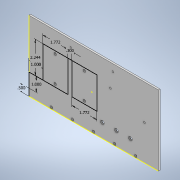
# Autodesk Inventor part: sheetmetalback2.0
Saved by Autodesk Inventor 2020.2 (Build 242310000, 310)
## iProperties
Created: 2020-02-06
Part Number: sheetmetalback2.0
Material: Generic
Document SubType Name: Sheet Metal
Designer: ColinP
Density: 1 g/cm^3
Sheet Metal Rule: Default
Appearance: Default
Author: ColinP
Autodesk Inventor part; units mm, degrees
ref_plane "YZ Plane" through (0, 0, 0) normal (1, 0, 0) x (0, 1, 0)
ref_plane "XZ Plane" through (0, 0, 0) normal (0, 1, 0) x (-1, 0, 0)
ref_plane "XY Plane" through (0, 0, 0) normal (0, 0, 1) x (1, 0, 0)
sketch "Sketch1" plane through (0, 0, 0) normal (0, 0, 1) x (1, 0, 0)
  line L0 (120.396, 63.5) -> (-114.3, 63.5)
  line L1 (-114.3, 63.5) -> (-114.3, -63.5)
  line L2 (-114.3, -63.5) -> (120.396, -63.5)
  line L3 (120.396, -63.5) -> (120.396, 63.5)
  point P0 (0, 0)
  dimension "d0" = 234.696
  dimension "d1" = 127
  measures "d0" distance of L2.end L1.end
  measures "d1" distance of L1.end L0.end
extrude "Plate1" add sketch "Sketch1" along normal blind 3.048
sketch "Sketch2" plane through (0, 0, 3.048) normal (0, 0, 1) x (1, 0, 0)
  line L0 (-114.3, 63.5) -> (-114.3, -63.5) projected
  line L1 (-114.3, -63.5) -> (-114.3, -60.325)
  line L2 (-114.3, -60.325) -> (-73.152, -60.325)
  line L3 (-73.152, -60.325) -> (-35.052, -60.325)
  line L4 (-35.052, -60.325) -> (3.048, -60.325)
  line L5 (3.048, -60.325) -> (41.148, -60.325)
  line L6 (41.148, -60.325) -> (79.248, -60.325)
  line L7 (79.248, -60.325) -> (120.396, -60.325)
  line L8 (120.396, -63.5) -> (120.396, 63.5) projected
  point P0 (0, 0)
  dimension "d3" = 3.175
  dimension "d4" = 41.148
  dimension "d5" = 38.1
  dimension "d6" = 38.1
  dimension "d7" = 38.1
  dimension "d8" = 38.1
  constraints: 14 end point, 6 point on line, 1 horizontal, 1 perpendicular
  measures "d3" distance of L0.end L1.end
  measures "d4" distance of L1.end L2.end
  measures "d5" distance of L2.end L3.end
  measures "d6" distance of L3.end L4.end
  measures "d7" distance of L4.end L5.end
  measures "d8" distance of L5.end L6.end
hole "Hole1" at (-73.152, -60.325, 3.048) at (-35.052, -60.325, 3.048) at (3.048, -60.325, 3.048) at (41.148, -60.325, 3.048) at (79.248, -60.325, 3.048) direction (0, 0, -1) diameter 4.4958 depth 3.048 clearance for "Hex Machine Screw" size "#8" standard "Ansi Unified Screw Threads"
sketch "Sketch3" plane through (0, 0, 3.048) normal (0, 0, 1) x (1, 0, 0)
  line L0 (-114.3, -63.5) -> (120.396, -63.5) projected
  line L1 (-114.3, -63.5) -> (-114.3, -50.8)
  line L2 (-114.3, 63.5) -> (-114.3, -63.5) projected
  line L3 (-114.3, -50.8) -> (-114.3, -25.4)
  line L4 (-114.3, -25.4) -> (-88.9, -25.4)
  line L5 (-88.9, -25.4) -> (-88.9, 31.6)
  line L6 (-88.9, 31.6) -> (-43.9, 31.6)
  line L7 (-43.9, 31.6) -> (-43.9, -25.4)
  line L8 (-43.9, -25.4) -> (-88.9, -25.4)
  line L9 (-43.9, 31.6) -> (-36.28, 31.6)
  line L10 (-36.28, 31.6) -> (-36.28, -25.4)
  line L11 (-36.28, -25.4) -> (8.72, -25.4)
  line L12 (8.72, -25.4) -> (8.72, 31.6)
  line L13 (8.72, 31.6) -> (-36.28, 31.6)
  point P0 (0, 0)
  dimension "d16" = 12.7
  dimension "d17" = 25.4
  dimension "d18" = 25.4
  dimension "d19" = 57
  dimension "d20" = 45
  dimension "d21" = 7.62
  dimension "d22" = 45
  constraints: 24 end point, 6 perpendicular, 6 point on line, 1 horizontal, 1 vertical
  measures "d16" distance of L0.start L1.end
  measures "d17" distance of L1.end L3.end
  measures "d18" distance of L3.end L4.end
  measures "d19" distance of L4.end L5.end
  measures "d20" distance of L5.end L6.end
  measures "d21" distance of L6.end L9.end
  measures "d22" distance of L10.end L11.end
sketch "Sketch4" plane through (0, 0, 3.048) normal (0, 0, 1) x (1, 0, 0)
  line L0 (-88.9, 31.6) -> (-43.9, 31.6) projected
  line L1 (-43.9, -25.4) -> (-88.9, -25.4) projected
  line L2 (-36.28, -25.4) -> (8.72, -25.4) projected
  line L3 (8.72, 31.6) -> (-36.28, 31.6) projected
  line L4 (-66.4, 31.6) -> (-66.4, 26.6)
  line L5 (-66.4, -25.4) -> (-66.4, -20.4)
  line L6 (-13.78, -25.4) -> (-13.78, -20.4)
  line L7 (-13.78, 31.6) -> (-13.78, 26.6)
  point P0 (0, 0)
  dimension "d23" = 5
  dimension "d24" = 5
  dimension "d25" = 5
  dimension "d26" = 5
  constraints: 8 end point, 4 midpoint, 4 vertical
  measures "d23" distance of L4.start L4.end
  measures "d24" distance of L5.start L5.end
  measures "d25" distance of L6.start L6.end
  measures "d26" distance of L7.start L7.end
hole "Hole2" at (-66.4, 26.6, 3.048) at (-66.4, -20.4, 3.048) at (-13.78, -20.4, 3.048) at (-13.78, 26.6, 3.048) direction (0, 0, -1) diameter 4.4958 depth 3.048 clearance for "Hex Machine Screw" size "#8" standard "Ansi Unified Screw Threads"
sketch "Sketch5" plane through (0, 0, 3.048) normal (0, 0, 1) x (1, 0, 0)
  line L0 (-114.3, -63.5) -> (120.396, -63.5) projected
  line L1 (120.396, -63.5) -> (120.396, -50.8)
  line L2 (120.396, -63.5) -> (120.396, 63.5) projected
  line L3 (120.396, -50.8) -> (120.396, 0)
  line L4 (120.396, 0) -> (94.996, 0)
  line L5 (94.996, 0) -> (94.996, 61.6)
  line L6 (94.996, 61.6) -> (71.996, 61.6)
  line L7 (8.72, -25.4) -> (8.72, 31.6) projected
  line L8 (94.996, 0) -> (33.396, 0)
  line L9 (33.396, 0) -> (33.396, 23)
  line L10 (94.996, 0) -> (94.996, 23)
  point P0 (0, 0)
  dimension "d34" = 12.7
  dimension "d35" = 50.8
  dimension "d36" = 25.4
  dimension "d37" = 61.6
  dimension "d38" = 23
  dimension "d46" = 61.6
  dimension "d47" = 23
  constraints: 16 end point, 4 perpendicular, 2 point on line, 1 horizontal, 1 midpoint
  measures "d34" distance of L0.end L1.end
  measures "d35" distance of L1.end L3.end
  measures "d36" distance of L3.end L4.end
  measures "d37" distance of L4.end L5.end
  measures "d38" distance of L5.end L6.end
  measures "d46" distance of L4.end L8.end
  measures "d47" distance of L8.end L9.end
hole "Hole3" at (33.396, 23, 3.048) at (94.996, 0, 3.048) direction (0, 0, -1) diameter 3.2766 depth 3.048 clearance for "Hex Machine Screw" size "#4" standard "Ansi Unified Screw Threads"
sketch "Sketch6" plane through (0, 0, 3.048) normal (0, 0, 1) x (1, 0, 0)
  line L0 (-114.3, -63.5) -> (-114.3, 63.5) projected
  line L1 (-114.3, 63.5) -> (-114.3, 50.8)
  line L2 (-114.3, 50.8) -> (-38.1, 50.8)
  line L3 (-38.1, 50.8) -> (38.1, 50.8)
  point P0 (0, 0)
  dimension "d48" = 12.7
  dimension "d49" = 76.2
  dimension "d50" = 76.2
  constraints: 6 end point, 2 point on line, 1 perpendicular
  measures "d48" distance of L0.end L1.end
  measures "d49" distance of L1.end L2.end
  measures "d50" distance of L2.end L3.end
hole "Hole4" at (-38.1, 50.8, 3.048) at (38.1, 50.8, 3.048) direction (0, 0, -1) diameter 3.2766 end through all clearance for "Flat Head Machine Screw (82)" size "#4" standard "Ansi Unified Screw Threads"
sketch "Sketch7" plane through (0, 0, 3.048) normal (0, 0, 1) x (1, 0, 0)
  line L0 (120.396, -63.5) -> (69.596, -63.5)
  line L1 (120.396, -63.5) -> (-114.3, -63.5) projected
  line L2 (69.596, -63.5) -> (69.596, -38.1)
  line L3 (69.596, -38.1) -> (44.196, -38.1)
  line L4 (44.196, -38.1) -> (18.796, -38.1)
  point P0 (0, 0)
  dimension "d58" = 50.8
  dimension "d59" = 25.4
  dimension "d60" = 25.4
  dimension "d61" = 25.4
  constraints: 8 end point, 2 perpendicular, 2 point on line
  measures "d58" distance of L0.start L0.end
  measures "d59" distance of L0.end L2.end
  measures "d60" distance of L2.end L3.end
  measures "d61" distance of L3.end L4.end
hole "Hole5" at (44.196, -38.1, 3.048) at (69.596, -38.1, 3.048) at (18.796, -38.1, 3.048) direction (0, 0, -1) diameter 6.7564 depth 3.048 clearance for "Flat Head Machine Screw (82)" size "1/4" standard "Ansi Unified Screw Threads"
equation "\"d14\" = Thickness"
equation "\"d32\" = Thickness"
equation "\"d44\" = Thickness"
equation "\"d56\" = Thickness"
equation "\"d67\" = Thickness"
equation "\"d2\" = Thickness"
equation "\"BendRadius\" = Thickness"
equation "\"BendReliefWidth\" = Thickness"
equation "\"BendReliefDepth\" = 0.5 * Thickness"
equation "\"CornerReliefSize\" = 4 * Thickness"
equation "\"MinimumRemnant\" = 2 * Thickness"
equation "\"TransitionRadius\" = BendRadius"
equation "\"JacobiRadiusSize\" = BendRadius"
equation "\"GapSize\" = Thickness"
equation "\"Thickness\" = 3.048"
body "Solid1"
